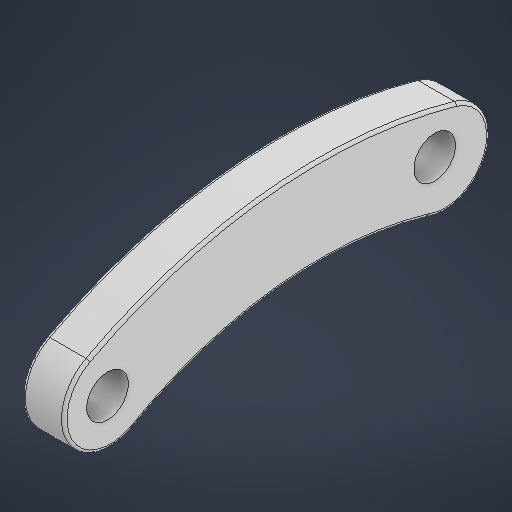
# Autodesk Inventor part: Lankarm_kort
Saved by Autodesk Inventor 2026 (Build 300175000, 175)
## iProperties
Created: 2025-04-29
Part Number: Lankarm_kort
Material: Generic
Document SubType Name: Modeling
Designer: elias
Density: 1 g/cm^3
Appearance: Default
Author: elias
Autodesk Inventor part; units mm, degrees
ref_plane "YZ Plane" through (0, 0, 0) normal (1, 0, 0) x (0, 1, 0)
ref_plane "XZ Plane" through (0, 0, 0) normal (0, 1, 0) x (-1, 0, 0)
ref_plane "XY Plane" through (0, 0, 0) normal (0, 0, 1) x (1, 0, 0)
sketch "Sketch1" plane through (0, 0, 0) normal (1, 0, 0) x (0, 1, 0)
  line L0 (2812.3869, 0) -> (2812.3869, -5171.1623) construction
  line L1 (2812.3869, -5171.1623) -> (0, -5171.1623) construction
  line L2 (0, -5171.1623) -> (0, 0) construction
  line L3 (0, 0) -> (2812.3869, 0) construction
  point P0 (0, 0)
  constraints: 2 end point, 2 other
sketch "Sketch2" plane through (0, 0, 0) normal (1, 0, 0) x (0, 1, 0)
  arc A0 (753.391, -1473.8258) -> (725.6652, -1208.6158) centre (409.0296, -1375.7721) ccw
  arc A1 (692.5478, -1452.6934) -> (667.2559, -1239.5627) centre (430.475, -1375.7271) ccw
  arc A2 (725.6652, -1208.6158) -> (667.2559, -1239.5627) centre (696.4374, -1224.0456) ccw
  arc A3 (692.5478, -1452.6934) -> (753.391, -1473.8258) centre (722.3676, -1464.9922) ccw
  circle A4 centre (696.4374, -1222.1798) radius 15
  circle A5 centre (727.5117, -1457.7884) radius 15
  point P0 (0, 0)
  dimension "d4" = 30
  dimension "d5" = 30
  constraints: 8 point on circle, 6 centre point, 2 tangent
  measures "d4" diameter of A4
  measures "d5" diameter of A5
extrude "Extrusion1" add sketch "Sketch2" along normal mid plane 30
fillet "Fillet1" radius 2 8 edges at (15, 765.1382, -1338.5435) (15, 680.964, -1194.8409) (15, 701.7128, -1343.5398) (15, 711.7843, -1495.4631) (-15, 765.1382, -1338.5435) (-15, 711.7843, -1495.4631) (-15, 701.7128, -1343.5398) (-15, 680.964, -1194.8409)
body "Solid1"
